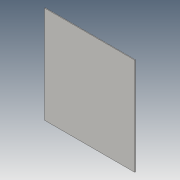
# Autodesk Inventor part: Bellypan
Saved by Autodesk Inventor 2016 (Build 200138000, 138)
## iProperties
Created: 2017-01-08
Part Number: Bellypan
Material: Generic
Document SubType Name: Modeling
Designer: idevr_000
Density: 1 g/cm^3
Appearance: Default
Author: idevr_000
Autodesk Inventor part; units mm, degrees
ref_plane "YZ Plane" through (0, 0, 0) normal (1, 0, 0) x (0, 1, 0)
ref_plane "XZ Plane" through (0, 0, 0) normal (0, 1, 0) x (-1, 0, 0)
ref_plane "XY Plane" through (0, 0, 0) normal (0, 0, 1) x (1, 0, 0)
sketch "Sketch1" plane through (0, 0, 0) normal (0, 0, 1) x (1, 0, 0)
  line L0 (-209.55, -225.425) -> (209.55, -225.425)
  line L1 (209.55, -225.425) -> (209.55, 225.425)
  line L2 (209.55, 225.425) -> (-209.55, 225.425)
  line L3 (-209.55, 225.425) -> (-209.55, -225.425)
  line L4 (-209.55, -225.425) -> (209.55, 225.425) construction
  line L5 (209.55, -225.425) -> (-209.55, 225.425) construction
  point P0 (0, 0)
  dimension "d0" = 419.1
  dimension "d1" = 450.85
  constraints: 12 end point, 2 midpoint, 2 parallel, 1 horizontal, 1 perpendicular
  measures "d0" distance of L2.end L1.end
  measures "d1" distance of L1.end L0.end
extrude "Extrusion1" add sketch "Sketch1" along normal blind 3.175
body "Solid1"
